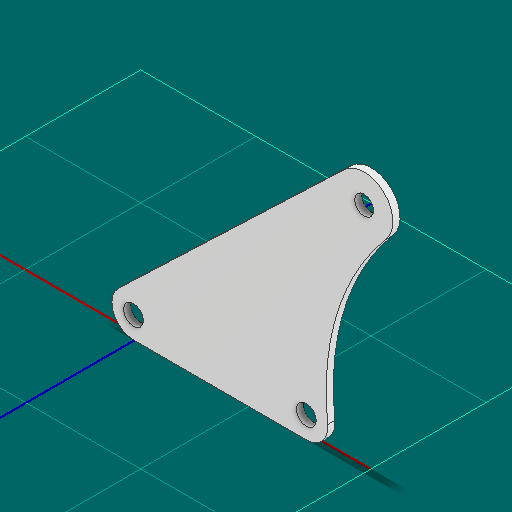
# Autodesk Inventor part: half_motor_mount
Saved by Autodesk Inventor 2025 (Build 290162000, 162)
## iProperties
Created: 2024-10-09
Part Number: half_motor_mount
Material: Acetal Resin, White
Document SubType Name: Modeling
Designer: averey
Density: 1.425 g/cm^3
Appearance: Smooth - White
Author: averey
Autodesk Inventor part; units mm, degrees
ref_plane "YZ Plane" through (0, 0, 0) normal (1, 0, 0) x (0, 1, 0)
ref_plane "XZ Plane" through (0, 0, 0) normal (0, 1, 0) x (-1, 0, 0)
ref_plane "XY Plane" through (0, 0, 0) normal (0, 0, 1) x (1, 0, 0)
sketch "main" plane through (0, 0, 0) normal (0, 0, 1) x (1, 0, 0)
  circle A0 centre (-26.3093, 39.0816) radius 2.1844
  circle A1 centre (-26.3093, 0.9816) radius 2.1844
  circle A2 centre (20.125, -11.7184) radius 2.0955
  arc A3 (15.9867, -16.5346) -> (24.712, -7.3272) centre (20.125, -11.7184) ccw
  arc A4 (-22.8691, 42.375) -> (-31.0718, 39.0816) centre (-26.3093, 39.0816) ccw
  line L0 (24.712, -7.3272) -> (-22.8691, 42.375)
  line L1 (-31.0718, 39.0816) -> (-31.0718, 0.9816)
  arc A5 (15.9867, -16.5346) -> (-25.7607, -3.7492) centre (-19.4895, -57.8222) ccw
  arc A6 (-31.0718, 0.9816) -> (-25.7607, -3.7492) centre (-26.3093, 0.9816) ccw
  point P0 (-11.6855, 6.8462)
  dimension "d0" = 4.191
  dimension "d1" = 50.8
  dimension "d2" = 12.7
  dimension "d3" = 9.525
  measures "d0" diameter of A2
  measures "d1" vertical distance of A0.centre A2.centre
  measures "d2" diameter of A3
  measures "d3" diameter of A4
sketch "Sketch1" plane through (0, 0, 0) normal (0, 0, 1) x (1, 0, 0)
  circle A0 centre (0, 0) radius 2.1844
  circle A1 centre (38.1, -0.042) radius 2.1844
  circle A2 centre (50.8511, 46.3784) radius 2.0955
  arc A3 (55.6628, 42.2347) -> (46.465, 50.9702) centre (50.8511, 46.3784) ccw
  arc A4 (-3.2896, 3.4438) -> (-0.0052, -4.7625) centre (0, 0) ccw
  line L0 (46.465, 50.9702) -> (-3.2896, 3.4438)
  line L1 (-0.0052, -4.7625) -> (38.0947, -4.8045)
  arc A5 (55.6628, 42.2347) -> (42.8314, 0.5015) centre (96.9113, 6.7131) ccw
  arc A6 (38.0947, -4.8045) -> (42.8314, 0.5015) centre (38.1, -0.042) ccw
  point P0 (0, 0)
  constraints: 1 other
extrude "Extrusion1" add sketch "Sketch1" along normal blind 1.5875
body "Solid1"
